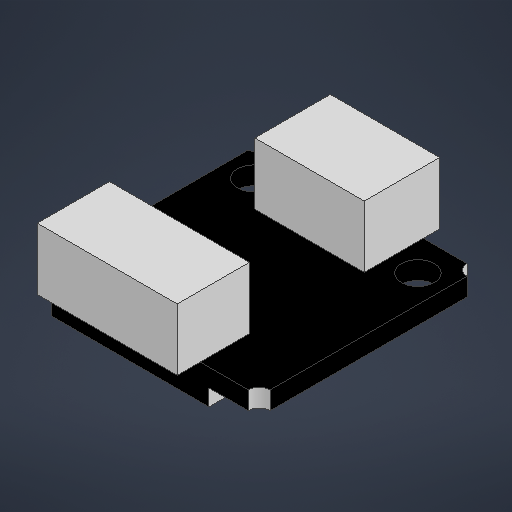
# Autodesk Inventor part: Limit Switch
Saved by Autodesk Inventor 2025.1 (Build 291241000, 241)
## iProperties
Created: 2025-03-05
Part Number: Limit Switch
Material: Generic
Document SubType Name: Modeling
Designer: jerem
Density: 1 g/cm^3
Appearance: Default
Author: jerem
Autodesk Inventor part; units mm, degrees
ref_plane "YZ Plane" through (0, 0, 0) normal (1, 0, 0) x (0, 1, 0)
ref_plane "XZ Plane" through (0, 0, 0) normal (0, 1, 0) x (-1, 0, 0)
ref_plane "XY Plane" through (0, 0, 0) normal (0, 0, 1) x (1, 0, 0)
sketch "Sketch1" plane through (0, 0, 0) normal (0, 1, 0) x (-1, 0, 0)
  line L0 (-10, -10) -> (10, -10)
  line L1 (10, -10) -> (10, 10)
  line L2 (10, 10) -> (-10, 10)
  line L3 (-10, 10) -> (-10, -10)
  line L4 (-10, -10) -> (10, 10) construction
  line L5 (10, -10) -> (-10, 10) construction
  circle A0 centre (7.5, -7) radius 1.5
  circle A1 centre (-7.5, -7) radius 1.5
  line L6 (7.5, -7) -> (-7.5, -7) construction
  line L7 (0, -7) -> (0, 0) construction
  dimension "d0" = 20
  dimension "d1" = 20
  dimension "d2" = 15
  dimension "d3" = 3
  dimension "d4" = 3
  constraints: 16 end point, 3 midpoint, 2 centre point, 2 horizontal, 2 parallel, 2 perpendicular, 1 equal radius
  measures "d0" distance of L2.end L1.end
  measures "d1" distance of L1.end L0.end
  measures "d2" distance of L6.start L6.end
  measures "d3" distance between parallel lines of L0 L6
  measures "d4" diameter of A0
extrude "Extrusion1" add sketch "Sketch1" along normal blind 1.65
sketch "Sketch2" plane through (0, 1.65, 0) normal (0, 1, 0) x (1, 0, 0)
  line L0 (-10, 10) -> (-10, -10) projected
  line L1 (-10, -10) -> (10, -10) projected
  line L2 (10, -10) -> (10, 10) projected
  line L3 (10, 10) -> (-10, 10) projected
  circle A0 centre (-7.5, 7) radius 1.5 projected
  circle A1 centre (7.5, 7) radius 1.5 projected
  line L4 (-5, 4.6) -> (5, 4.6)
  line L5 (5, 4.6) -> (5, 11.5)
  line L6 (5, 11.5) -> (-5, 11.5)
  line L7 (-5, 11.5) -> (-5, 4.6)
  line L8 (0, 4.6) -> (0, 0) construction
  point P0 (5, 10)
  point P1 (-5, 10)
  dimension "d7" = 10
  dimension "d8" = 6.9
  dimension "d9" = 1.5
  constraints: 10 end point, 2 parallel, 2 perpendicular, 1 horizontal, 1 midpoint
  measures "d7" distance of L5.end L6.end
  measures "d8" distance of L6.end L4.start
  measures "d9" distance between parallel lines of L3 L6
extrude "Extrusion2" add sketch "Sketch2" along normal blind 5.65 contours L7 L6 L5 L3 | L3 L5 L4 L7
sketch "Sketch3" plane through (0, 1.65, 0) normal (0, 1, 0) x (1, 0, 0)
  line L0 (-8.2, -12.1) -> (4.6, -12.1)
  line L1 (4.6, -12.1) -> (4.6, -5.5)
  line L2 (4.6, -5.5) -> (-8.2, -5.5)
  line L3 (-8.2, -5.5) -> (-8.2, -12.1)
  line L4 (-10, 10) -> (-10, -10) projected
  line L5 (-10, -10) -> (10, -10) projected
  point P0 (0, 0)
  dimension "d12" = 1.8
  dimension "d13" = 12.8
  dimension "d14" = 6.6
  dimension "d15" = 2.1
  constraints: 8 end point, 2 parallel, 1 horizontal, 1 perpendicular
  measures "d12" distance between parallel lines of L4 L3
  measures "d13" distance of L0.start L0.end
  measures "d14" distance of L0.end L1.end
  measures "d15" distance between parallel lines of L5 L0
extrude "Extrusion3" add sketch "Sketch3" along normal blind 5.65
fillet "Fillet1" radius 1 4 edges at (10, 0.825, 10) (10, 0.825, -10) (-10, 0.825, 10) (-10, 0.825, -10) inverted yes
sketch "Sketch4" plane through (0, 0, 0) normal (0, -1, 0) x (1, 0, 0)
  line L0 (3.8, -4.6) -> (-2.4, -4.6)
  line L1 (-2.4, -4.6) -> (-2.4, -5.6)
  line L2 (-2.4, -5.6) -> (3.8, -5.6)
  line L3 (3.8, -5.6) -> (3.8, -4.6)
  line L4 (10, 9) -> (10, -9) projected
  line L5 (9, -10) -> (-9, -10) projected
  line L6 (-9, 10) -> (9, 10) projected
  arc A0 (-10, 9) -> (-9, 10) centre (-10, 10) ccw projected
  line L7 (-10, -9) -> (-10, 9) projected
  line L8 (5.4, 10) -> (5.4, 1.8)
  line L9 (5.4, 1.8) -> (-10, 1.8)
  point P0 (0, 0)
  dimension "d19" = 6.2
  dimension "d20" = 6.2
  dimension "d21" = 4.4
  dimension "d22" = 1
  dimension "d23" = 4.6
  dimension "d24" = 8.2
  constraints: 12 end point, 2 parallel, 2 perpendicular, 2 point on line, 1 horizontal, 1 vertical
  measures "d19" distance of L0.start L0.end
  measures "d20" distance between parallel lines of L4 L3
  measures "d21" distance between parallel lines of L5 L2
  measures "d22" distance of L0.end L1.end
  measures "d23" distance between parallel lines of L4 L8
  measures "d24" distance between parallel lines of L6 L9
extrude "Extrusion4" add sketch "Sketch4" along normal blind 1.5
shell "Shell1" thickness 1 removed faces 1 at (1.6667, 3.5333, -11.5)
body "Solid1"
